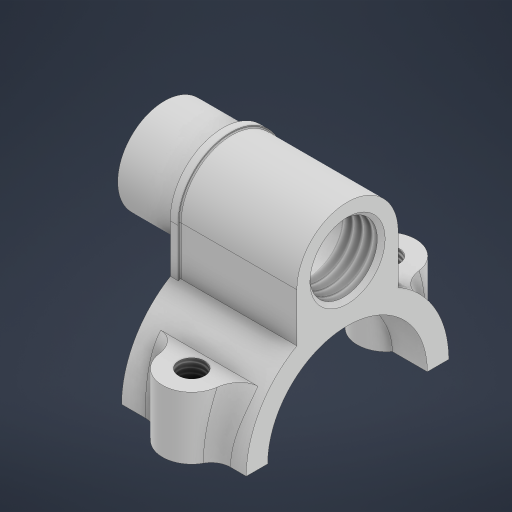
# Autodesk Inventor part: Part5
Saved by Autodesk Inventor 2023 (Build 270158000, 158)
## iProperties
Created: 2023-04-26
Part Number: Part5
Material: Ogólny
Document SubType Name: Modeling
Designer: Adam
Density: 1 g/cm^3
Appearance: Domyślna
Author: Adam
Autodesk Inventor part; units mm, degrees
ref_plane "YZ Plane" through (0, 0, 0) normal (1, 0, 0) x (0, 1, 0)
ref_plane "XZ Plane" through (0, 0, 0) normal (0, 1, 0) x (-1, 0, 0)
ref_plane "XY Plane" through (0, 0, 0) normal (0, 0, 1) x (1, 0, 0)
sketch "Szkic1" plane through (0, 0, 0) normal (1, 0, 0) x (0, 1, 0)
  arc A0 (0, -20.5) -> (0, 20.5) centre (0, 0) ccw
  arc A1 (0, -26) -> (0, 26) centre (0, 0) ccw
  line L0 (0, 26) -> (0, 20.5)
  line L1 (0, -20.5) -> (0, -26)
  circle A2 centre (35, 0) radius 13
  line L2 (35, 13) -> (22.5167, 13)
  line L3 (35, -13) -> (22.5167, -13)
  dimension "d2" = 26
  dimension "d3" = 20.5
  dimension "d5" = 26
  constraints: 8 end point, 8 point on circle, 3 centre point, 2 coincident, 2 equal length, 2 tangent, 1 horizontal, 1 vertical
  measures "d2" radius of A1
  measures "d3" radius of A0
  measures "d5" diameter of A2
extrude "Wyciągnięcie proste1" add sketch "Szkic1" along normal mid plane 30
sketch "Szkic3" plane through (-15, 0, 0) normal (-1, 0, 0) x (0, 0, 1)
  arc A0 (13.4871, 34.5452) -> (-13.4936, 34.4383) centre (-0.0053, 35) ccw
  line L0 (-13.4936, 34.4383) -> (-13.4936, 22.2244)
  arc A1 (-13, 22.5167) -> (-26, 0) centre (0, 0) ccw projected
  line L1 (13.4871, 34.5452) -> (13.4871, 22.2283)
  arc A2 (26, 0) -> (13, 22.5167) centre (0, 0) ccw projected
  arc A3 (-13.4936, 22.2244) -> (-26, 0) centre (0, 0) ccw
  arc A4 (26, 0) -> (13.4871, 22.2283) centre (0, 0) ccw
  arc A5 (20.5, 0) -> (-20.5, 0) centre (0, 0) ccw projected
  arc A6 (20.5, 0) -> (-20.5, 0) centre (0, 0) ccw
  line L2 (-20.5, 0) -> (-26, 0) projected
  line L3 (-26, 0) -> (-20.5, 0)
  line L4 (-20.5, 0) -> (-26, 0)
  line L5 (26, 0) -> (20.5, 0) projected
  line L6 (20.5, 0) -> (26, 0)
  line L7 (26, 0) -> (20.5, 0)
  line L8 (-20.5, 0) -> (-26, 0)
  line L9 (20.5, 0) -> (26, 0)
  dimension "d18" = 13.5
  dimension "d22" = 35
  constraints: 16 end point, 10 point on circle, 4 centre point, 3 coincident, 3 collinear, 1 parallel, 1 vertical
  measures "d18" radius of A0
  measures "d22" distance of point (0, 0) A0.centre
extrude "Wyciągnięcie proste2" add sketch "Szkic3" along normal blind 2
fillet "Zaokrąglenie powierzchni2" radius 0.268 1 edges at (-15, 48, 0)
sketch "Szkic4" plane through (-17, 0, 0) normal (-1, 0, 0) x (0, 0, 1)
  circle A0 centre (0, 35) radius 12
  point P0 (0, 0)
  dimension "d24" = 24
  constraints: 1 centre point, 1 coincident
  measures "d24" diameter of A0
extrude "Wyciągnięcie proste3" add sketch "Szkic4" along normal blind 15
sketch "Szkic5" plane through (15, 0, 0) normal (1, 0, 0) x (0, 0, -1)
  point P0 (0, 0)
  point P1 (0, 35)
hole "Otwór2" at (15, 35, 0) direction (-1, 0, 0) diameter 17.294 end through all thread size "M20x2.5" class "6H" standard "ANSI Metric M Profile"
chamfer "Faza2" distance 1 angle 45 1 edges at (-32, 35, 8.647) measured on face at (-32, 35, 9.147)
chamfer "Faza3" distance 1 angle 45 1 edges at (15, 35, 8.647) measured on face at (15, 35, 9.147)
sketch "Szkic6" plane through (0, 0, 0) normal (0, 0, 1) x (1, 0, 0)
  point P0 (0, 0)
sketch "Szkic7" plane through (0, 0, 0) normal (0, 1, 0) x (-1, 0, 0)
  point P0 (0, 0)
sketch "Szkic8" plane through (0, 0, 0) normal (0, 1, 0) x (-1, 0, 0)
  line L0 (-15, -26) -> (-15, -20.5) projected
  line L1 (-15, -20.5) -> (17, -20.5) projected
  line L2 (17, -20.5) -> (17, -26) projected
  line L3 (17, -26) -> (-15, -26) projected
  line L4 (17, 26) -> (17, 20.5) projected
  line L5 (17, 20.5) -> (-15, 20.5) projected
  line L6 (-15, 20.5) -> (-15, 26) projected
  line L7 (-15, 26) -> (17, 26) projected
  circle A0 centre (0, 0) radius 5
  dimension "d40" = 10
  constraints: 1 centre point, 1 coincident
  measures "d40" diameter of A0
extrude "Wyciągnięcie proste4" add sketch "Szkic8" along normal up to next contours A0
sketch "Szkic9" plane through (0, 0, 0) normal (0, -1, 0) x (1, 0, 0)
  circle A0 centre (0, 0) radius 5
  constraints: 1 centre point, 1 coincident
extrude "Wyciągnięcie proste5" cut sketch "Szkic9" against normal blind 15
chamfer "Faza4" distance 0.5 angle 45 1 edges at (5, 15, 0) measured on face at (4.5, 15, 0)
fillet "Zaokrąglenie powierzchni3" radius 0.5 1 edges at (5, 20.5, 0)
sketch "Szkic10" plane through (0, 0, 0) normal (0, 1, 0) x (-1, 0, 0)
  circle A0 centre (0, 25) radius 7.5
  circle A1 centre (0, -25) radius 7.5
  point P0 (0, 0)
  dimension "d49" = 15
  dimension "d50" = 15
  constraints: 2 centre point
  measures "d49" diameter of A0
  measures "d50" diameter of A1
extrude "Wyciągnięcie proste6" add sketch "Szkic10" along normal blind 16
fillet "Zaokrąglenie1" radius 5 6 edges at (-7.4623, 3.5887, 25.7511) (-7.2751, 11.7824, 23.177) (7.4905, 8.3515, 24.6222) (7.4905, 8.3514, -24.6222) (-7.2749, 11.7839, -23.1763) (-7.4623, 3.5887, -25.7511)
sketch "Szkic11" plane through (15, 0, -26) normal (0, -1, 0) x (1, 0, 0)
  arc A0 (-9, 5.5) -> (-21, 5.5) centre (-15, 1) ccw projected
  arc A1 (-8.4205, 54.6) -> (-21.5795, 54.6) centre (-15, 51) ccw projected
  point P0 (-15, 26)
  constraints: 2 coincident
hole "Otwór3" at (0, 0, -25) at (0, 0, 25) direction (0, 1, 0) diameter 6.647 end through all thread size "M8x1.25" class "6H" standard "ANSI Metric M Profile"
chamfer "Faza5" distance 0.75 angle 45 1 edges at (0, 0, -21.6765) measured on face at (0, 0, -21.1765)
chamfer "Faza6" distance 0.75 angle 45 1 edges at (0, 0, 28.3235) measured on face at (0, 0, 28.8235)
